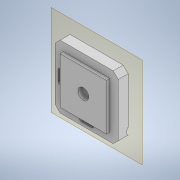
# Autodesk Inventor part: 20_Cube_Insert_Kinematic_Beautymirrormount_90_pro_v3
Saved by Autodesk Inventor 2022 (Build 260153000, 153)
## iProperties
Created: 2021-11-15
Part Number: 20_Cube_Insert_Kinematic_Beautymirrormount_90_pro_v3
Material: Generic
Document SubType Name: Modeling
Designer: diederichbenedict
Density: 1 g/cm^3
Appearance: Default
Author: diederichbenedict
Autodesk Inventor part; units mm, degrees
ref_plane "YZ Plane" through (0, 0, 0) normal (1, 0, 0) x (0, 1, 0)
ref_plane "XZ Plane" through (0, 0, 0) normal (0, 1, 0) x (-1, 0, 0)
ref_plane "XY Plane" through (0, 0, 0) normal (0, 0, 1) x (1, 0, 0)
ref_plane "Work Plane1" through (0, 0, 2) normal (0, 0, 1) x (1, 0, 0)
sketch "Sketch1" plane through (0, 0, 2) normal (0, 0, 1) x (1, 0, 0)
  circle A0 centre (-37.0712, 14) radius 3.25 construction
  circle A1 centre (-9.0712, -14) radius 3.25 construction
  line L0 (-26.0712, -17.08) -> (-20.0712, -17.08) construction
  arc A2 (-20.0712, -17.08) -> (-20.0712, -14.08) centre (-20.0712, -15.58) ccw construction
  line L1 (-20.0712, -14.08) -> (-26.0712, -14.08) construction
  line L2 (-37.0712, -3) -> (-37.0712, 3) construction
  arc A3 (-37.0712, 3) -> (-40.0712, 3) centre (-38.5712, 3) ccw construction
  line L3 (-40.0712, 3) -> (-40.0712, -3) construction
  line L4 (-47.9712, -17) -> (-47.9712, 17) construction
  line L5 (-47.9712, 17) -> (-44.3964, 17) construction
  line L6 (-44.3964, 17) -> (-40.0712, 21.3252) construction
  line L7 (-40.0712, 21.3252) -> (-40.0712, 24.9) construction
  line L8 (-40.0712, 24.9) -> (-6.0712, 24.9) construction
  line L9 (-6.0712, 24.9) -> (-6.0712, 21.3252) construction
  line L10 (-6.0712, 21.3252) -> (-1.746, 17) construction
  line L11 (-1.746, 17) -> (1.8288, 17) construction
  line L12 (1.8288, 17) -> (1.8288, -17) construction
  line L13 (1.8288, -17) -> (-1.746, -17) construction
  line L14 (-1.746, -17) -> (-6.1126, -21.3666) construction
  line L15 (-6.1126, -21.3666) -> (-6.1126, -24.9) construction
  line L16 (-6.1126, -24.9) -> (-40.0712, -24.9) construction
  circle A4 centre (-37.0712, -14) radius 3.25 construction
  circle A5 centre (-23.0712, 0) radius 12.45 construction
  circle A6 centre (-23.0712, 0) radius 12.7 construction
  line L17 (-37.0712, 14) -> (-9.0712, 14) construction
  line L18 (-9.0712, 14) -> (-9.0712, -14) construction
  line L19 (-9.0712, -14) -> (-37.0712, -14) construction
  line L20 (-37.0712, -14) -> (-37.0712, 14) construction
  line L21 (-4.0712, -19) -> (-4.0712, 19)
  line L22 (-4.0712, 19) -> (-42.0712, 19)
  line L23 (-42.0712, 19) -> (-42.0712, -19)
  line L24 (-42.0712, -19) -> (-4.0712, -19)
  circle A7 centre (-23.0712, 0) radius 12.8
  circle A8 centre (-23.0712, 0) radius 3.25 projected
  line L25 (-40.0712, -24.9) -> (-40.0712, -21.3252) projected
  line L26 (-40.0712, -21.3252) -> (-44.3964, -17) projected
  line L27 (-44.3964, -17) -> (-47.9712, -17) projected
  arc A9 (-26.0712, -14.08) -> (-26.0712, -17.08) centre (-26.0712, -15.58) ccw projected
  arc A10 (-40.0712, -3) -> (-37.0712, -3) centre (-38.5712, -3) ccw projected
  circle A11 centre (-37.0712, -14) radius 3.25 projected
  point P0 (0, 0)
  point P1 (-21.8762, -3.0223)
  point P2 (-25.9925, 1.4242)
  dimension "d0" = 5
  dimension "d1" = 0.1
  constraints: 16 end point, 4 parallel, 2 perpendicular, 1 centre point, 1 horizontal, 3 other
  measures "d0" distance between parallel lines of L18 L21
  measures "d1" radial gap between concentric circles of A6 A7
extrude "Extrusion1" add sketch "Sketch1" along normal blind 6 contours L24 L23 L22 L21 | A7 | A11
sketch "Sketch2" plane through (0, 0, 2) normal (0, 0, -1) x (-1, 0, 0)
  circle A0 centre (23.0712, 0) radius 12.8 projected
  circle A1 centre (23.0712, 0) radius 8.5824
  point P0 (0, 0)
  constraints: 1 centre point
extrude "Extrusion2" add sketch "Sketch2" against normal blind 0.5
sketch "Sketch3" plane through (0, 0, 2) normal (0, 0, -1) x (-1, 0, 0)
  circle A0 centre (9.0712, -14) radius 1.45 construction
  circle A1 centre (9.0712, -14) radius 2.45
  circle A2 centre (37.0712, -14) radius 1.45 projected
  circle A3 centre (37.0712, -14) radius 1.95
  point P0 (0, 0)
  dimension "d8" = 1
  dimension "d10" = 0.5
  constraints: 2 centre point
  measures "d8" radial gap between concentric circles of A0 A1
  measures "d10" radial gap between concentric circles of A2 A3
sketch "Sketch5" plane through (0, 0, 2) normal (0, 0, -1) x (-1, 0, 0)
  arc A0 (20.0712, -14.08) -> (20.0712, -17.08) centre (20.0712, -15.58) ccw projected
  arc A1 (26.0712, -17.08) -> (26.0712, -14.08) centre (26.0712, -15.58) ccw projected
  line L0 (37.0712, 3) -> (37.0712, -3) projected
  arc A2 (37.0712, -3) -> (40.0712, -3) centre (38.5712, -3) ccw projected
  line L1 (40.0712, -3) -> (40.0712, 3) projected
  arc A3 (40.0712, 3) -> (37.0712, 3) centre (38.5712, 3) ccw projected
  line L2 (26.0712, -14.08) -> (20.0712, -14.08) projected
  arc A4 (20.0712, -14.08) -> (20.0712, -17.08) centre (20.0712, -15.58) ccw projected
  line L3 (20.0712, -17.08) -> (26.0712, -17.08) projected
  arc A5 (26.0712, -17.08) -> (26.0712, -14.08) centre (26.0712, -15.58) ccw projected
  circle A6 centre (37.0712, -14) radius 1.45 projected
  circle A7 centre (23.0712, 0) radius 1.45 projected
  circle A8 centre (9.0712, -14) radius 1.45 projected
  circle A9 centre (37.0712, 14) radius 1.45 projected
  line L4 (-1.8288, -17) -> (-1.8288, 17) projected
  line L5 (-1.8288, 17) -> (1.746, 17) projected
  line L6 (1.746, 17) -> (6.0712, 21.3252) projected
  line L7 (6.0712, 21.3252) -> (6.0712, 24.9) projected
  line L8 (6.0712, 24.9) -> (40.0712, 24.9) projected
  line L9 (40.0712, 24.9) -> (40.0712, 21.3252) projected
  line L10 (40.0712, 21.3252) -> (44.3964, 17) projected
  line L11 (44.3964, 17) -> (47.9712, 17) projected
  line L12 (47.9712, 17) -> (47.9712, -17) projected
  line L13 (44.3964, -17) -> (47.9712, -17) projected
  line L14 (40.0712, -21.3252) -> (44.3964, -17) projected
  line L15 (40.0712, -24.9) -> (40.0712, -21.3252) projected
  line L16 (6.1126, -24.9) -> (40.0712, -24.9) projected
  line L17 (6.1126, -24.9) -> (6.1126, -21.3666) projected
  line L18 (6.1126, -21.3666) -> (1.746, -17) projected
  line L19 (1.746, -17) -> (-1.8288, -17) projected
  point P0 (0, 0)
  point P1 (40.0712, -3)
extrude "Extrusion5" cut sketch "Sketch5" against normal blind 8 contours L2 A1 L3 A0 | A3 L1 A2 L0
sketch "Sketch6" plane through (-42.0712, -19, 8) normal (0, -1, 0) x (1, 0, 0)
  line L0 (0, -6) -> (38, -6) projected
  line L1 (38, -6) -> (38, 0) projected
  line L2 (0, 0) -> (38, 0) projected
  line L3 (0, -6) -> (0, 0) projected
  line L4 (31.8, 0) -> (31.8, 0) projected
  circle A0 centre (19, -3) radius 1.45
  point P0 (42.0712, -8)
  point P1 (4.5, 0)
  dimension "d34" = 2.9
  constraints: 1 centre point
  measures "d34" diameter of A0
extrude "Extrusion6" cut sketch "Sketch6" against normal blind 8 contours A0
pattern_circular "Circular Pattern1" count 2 over 90 about axis through (-23.0712, 0, 2) along (0, 0, -1) of "Extrusion6"
chamfer "Chamfer1" distance 3 angle 45 4 edges at (-42.0712, 19, 5) (-4.0712, 19, 5) (-4.0712, -19, 5) (-42.0712, -19, 5)
hole "Hole1" at (-37.0712, -14, 2) direction (0, 0, 1) diameter 4 depth 0.1 tip angle 115
sketch "Sketch4" plane through (-4.0712, -19, 2) normal (1, 0, 0) x (0, 0, -1)
  line L0 (2, 4.45) -> (6, 4.45)
  line L1 (2, 1.55) -> (6, 1.55)
  line L2 (0, 0) -> (0, 38) projected
  arc A0 (2, 19) -> (2, 19) centre (1.5, 4.4206) ccw projected
  line L3 (-1.3741, 5) -> (-0.1, 7) projected
  line L4 (-1.3741, 5) -> (-0.1, 3) projected
  line L5 (-0.1, 7) -> (0.6045, 7)
  line L6 (0.6045, 7) -> (0.6045, 3)
  line L7 (0.6045, 3) -> (-0.1, 3)
  line L8 (-0.1, 3) -> (-0.1, 7)
  constraints: 12 end point, 3 horizontal, 2 parallel, 1 perpendicular, 4 other
extrude "Extrusion4" cut sketch "Sketch4" against normal blind 8 contours L7 L8 L5 L2 | L2 L5 L6 L7 | L4 L3 L8
sketch "Skizze8" plane through (0, 0, 8) normal (0, 0, 1) x (1, 0, 0)
  line L0 (-39.0712, -19) -> (-42.0712, -16) projected
  line L1 (-39.0712, -19) -> (-7.0712, -19) projected
  line L2 (-4.0712, -16) -> (-7.0712, -19) projected
  line L3 (-4.0712, -16) -> (-4.0712, 16) projected
  line L4 (-7.0712, 19) -> (-4.0712, 16) projected
  line L5 (-7.0712, 19) -> (-39.0712, 19) projected
  line L6 (-42.0712, 16) -> (-39.0712, 19) projected
  line L7 (-42.0712, 16) -> (-42.0712, -16) projected
  arc A0 (-37.0712, 3) -> (-40.0712, 3) centre (-38.5712, 3) ccw projected
  line L8 (-37.0712, 3) -> (-37.0712, -3) projected
  arc A1 (-40.0712, -3) -> (-37.0712, -3) centre (-38.5712, -3) ccw projected
  line L9 (-40.0712, -3) -> (-40.0712, 3) projected
  line L10 (-20.0712, -17.08) -> (-26.0712, -17.08) projected
  arc A2 (-26.0712, -14.08) -> (-26.0712, -17.08) centre (-26.0712, -15.58) ccw projected
  line L11 (-26.0712, -14.08) -> (-20.0712, -14.08) projected
  arc A3 (-20.0712, -17.08) -> (-20.0712, -14.08) centre (-20.0712, -15.58) ccw projected
  circle A4 centre (-23.0712, 0) radius 3.25 projected
  line L12 (-9.0712, -14) -> (-37.0712, -14)
  line L13 (-37.0712, -14) -> (-37.0712, 14)
  line L14 (-37.0712, 14) -> (-9.0712, 14)
  line L15 (-9.0712, 14) -> (-9.0712, -14)
  line L16 (-9.0712, -14) -> (-37.0712, 14) construction
  line L17 (-37.0712, -14) -> (-9.0712, 14) construction
  point P0 (0, 0)
  constraints: 12 end point, 2 midpoint, 2 parallel, 1 horizontal, 1 perpendicular
extrude "Extrusion8" add sketch "Skizze8" along normal blind 2 contours L13 L14 L15 L12 L8
body "Solid1"
